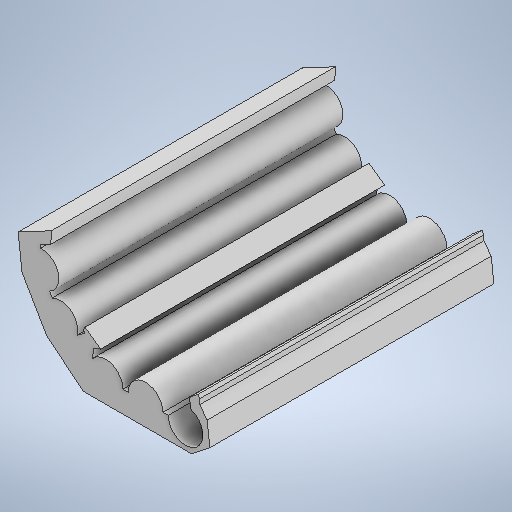
# Autodesk Inventor part: battery_case
Saved by Autodesk Inventor 2025.2 (Build 292293000, 293)
## iProperties
Created: 2025-03-06
Part Number: battery_case
Material: Generic
Document SubType Name: Modeling
Designer: aaron
Density: 1 g/cm^3
Appearance: Default
Author: aaron
Autodesk Inventor part; units mm, degrees
ref_plane "YZ Plane" through (0, 0, 0) normal (1, 0, 0) x (0, 1, 0)
ref_plane "XZ Plane" through (0, 0, 0) normal (0, 1, 0) x (-1, 0, 0)
ref_plane "XY Plane" through (0, 0, 0) normal (0, 0, 1) x (1, 0, 0)
sketch "Sketch1" plane through (0, 0, 0) normal (0, 0, 1) x (1, 0, 0)
  circle A0 centre (-37.5637, 37.4433) radius 13
  line L0 (-37.5637, 37.4433) -> (-3.6418, 16.2465)
  circle A1 centre (-3.6418, 16.2465) radius 13
  line L1 (-3.6418, 16.2465) -> (26.3582, 16.2465)
  circle A2 centre (26.3582, 16.2465) radius 13
  line L2 (26.3582, 16.2465) -> (56.3582, 16.2465)
  circle A3 centre (56.3582, 16.2465) radius 13
  line L3 (-37.5637, 37.4433) -> (-51.6479, 63.9317)
  circle A4 centre (-51.6479, 63.9317) radius 13
  line L4 (0, 0) -> (60.815, 0)
  line L5 (0, 0) -> (-20.4868, 0)
  line L6 (-20.4868, 0) -> (-48.0374, 22.6897)
  line L7 (-48.0374, 22.6897) -> (-66.3867, 54.4717)
  line L8 (-66.3867, 54.4717) -> (-69.1774, 79.0756)
  line L9 (60.815, 0) -> (74.4958, 10.7752)
  line L10 (74.4958, 10.7752) -> (72.5664, 27.7853)
  line L11 (72.5664, 27.7853) -> (66.9442, 34.9236)
  line L12 (-52.7512, 79.1009) -> (-52.443, 76.9074)
  line L13 (-44.4918, 53.0786) -> (-42.5598, 49.4449)
  line L14 (9.276, 17.7056) -> (13.4403, 17.7056)
  line L15 (39.276, 17.7056) -> (43.4403, 17.7056)
  line L16 (-25.0241, 34.0142) -> (-19.2859, 38.2885)
  line L17 (-19.2859, 38.2885) -> (-20.0356, 40.1123)
  line L18 (-20.0356, 40.1123) -> (-19.0512, 42.2941)
  line L19 (-19.0512, 42.2941) -> (-7.3799, 33.8874)
  line L20 (-7.3799, 33.8874) -> (-12.491, 31.9162)
  line L21 (-12.491, 31.9162) -> (-13.4773, 24.7473)
  line L22 (66.9442, 34.9236) -> (66.9442, 38.8151)
  line L23 (66.9442, 38.8151) -> (65.6719, 41.0187)
  line L24 (65.6719, 41.0187) -> (59.2097, 35.8187)
  line L25 (59.2097, 35.8187) -> (60.4815, 28.5753)
  line L26 (-69.1774, 79.0756) -> (-44.3667, 92.2677)
  line L27 (-44.3667, 92.2677) -> (-44.6875, 83.3885)
  line L28 (-44.6875, 83.3885) -> (-52.7512, 79.1009)
  point P0 (43.3582, 16.2465)
  point P1 (39.3582, 16.2465)
  point P2 (13.3582, 16.2465)
  point P3 (9.3582, 16.2465)
  point P4 (-14.6664, 23.1355)
  point P5 (-26.5391, 30.5544)
  point P6 (-43.6669, 48.9216)
  point P7 (-45.5448, 52.4534)
  point P8 (-57.5412, 70.4262)
  point P9 (-46.5604, 46.2337)
  point P10 (-56.0607, 64.118)
  point P11 (-36.7363, 29.1915)
  point P12 (-3.6418, 16.2465)
  dimension "d0" = 26
  dimension "d1" = 40
  dimension "d2" = 26
  dimension "d3" = 30
  dimension "d4" = 26
  dimension "d5" = 30
  dimension "d6" = 26
  dimension "d7" = 30
  dimension "d8" = 26
  dimension "d11" = 148
  dimension "d12" = 150
  constraints: 59 end point, 10 point on circle, 5 centre point, 4 parallel, 2 coincident, 2 horizontal, 2 point on line, 1 perpendicular, 1 vertical
  measures "d0" diameter of A0
  measures "d1" distance of L0.start L0.end
  measures "d2" diameter of A1
  measures "d3" distance of L1.end L1.start
  measures "d4" diameter of A2
  measures "d5" distance of L1.end L2.end
  measures "d6" diameter of A3
  measures "d7" distance of L3.end L0.start
  measures "d8" diameter of A4
  measures "d11" angle of L0 L1
  measures "d12" angle of L3 L0
extrude "Extrusion1" add sketch "Sketch1" along normal blind 213 contours A0 L0 L3 | L16 L17 L18 L19 L20 L21 A1 L0 A0 | L3 L0 A0 | A0 L0 A1 L1 A2 L2 A3 L25 L24 L23 L22 L11 L10 L9 L4 L5 L6 L7 L8 L26 L27 L28 L12 A4 L3 | A4 | A1 L1 L0 | L0 L1 A1 | A2 L2 L1 | L1 L2 A2
equation "\"d2\" = d0"
equation "\"d3\" = d5"
equation "\"d4\" = d0"
equation "\"d6\" = d0"
equation "\"d7\" = d5"
equation "\"d8\" = d0"
body "Solid1"
